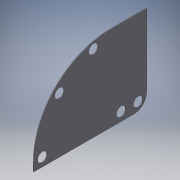
# Autodesk Inventor part: waterjet wall
Saved by Autodesk Inventor 2018 (Build 220112000, 112)
## iProperties
Created: 2020-01-24
Part Number: waterjet wall
Material: Generic
Document SubType Name: Modeling
Designer: s-2513225
Density: 1 g/cm^3
Appearance: Default
Author: s-2513225
Autodesk Inventor part; units mm, degrees
ref_plane "YZ Plane" through (0, 0, 0) normal (1, 0, 0) x (0, 1, 0)
ref_plane "XZ Plane" through (0, 0, 0) normal (0, 1, 0) x (-1, 0, 0)
ref_plane "XY Plane" through (0, 0, 0) normal (0, 0, 1) x (1, 0, 0)
sketch "Sketch1" plane through (0, 0, 0) normal (1, 0, 0) x (0, 1, 0)
  line L0 (-88.9, 0) -> (88.9, 0) construction
  line L1 (88.9, 0) -> (117.4115, 0) construction
  line L2 (165.1, -128.3993) -> (165.1, -77.5993)
  line L3 (-63.5, 151.0007) -> (-88.9, 151.0007)
  line L4 (-88.9, 151.0007) -> (-63.5, 151.0007) construction
  line L5 (-63.5, 151.0007) -> (-63.5, 125.6007) construction
  circle A0 centre (-63.5, 125.6007) radius 14.2875
  line L6 (-63.5, 125.6007) -> (-63.5, -26.7993) construction
  line L7 (-63.5, -26.7993) -> (139.7, -26.7993) construction
  circle A1 centre (139.7, -26.7993) radius 14.2875
  line L8 (-63.5, 125.6007) -> (76.2, 125.6007) construction
  line L9 (76.2, 125.6007) -> (76.2, 74.8007) construction
  circle A2 centre (76.2, 74.8007) radius 14.2875
  line L10 (-50.8, -185.5493) -> (165.1, -185.5493)
  line L11 (165.1, -185.5493) -> (165.1, -128.3993)
  arc A3 (165.1, -77.5993) -> (-63.5, 151.0007) centre (-63.5, -77.5993) ccw
  line L12 (-88.9, -147.4493) -> (-88.9, 151.0007)
  arc A4 (-88.9, -147.4493) -> (-50.8, -185.5493) centre (-50.8, -147.4493) ccw
  point P0 (0, 0)
  point P1 (165.1, 151.0007)
  point P2 (-88.9, -185.5493)
  dimension "d2" = 28.5115
  dimension "d5" = 279.4
  dimension "d8" = 25.4
  dimension "d9" = 25.4
  dimension "d10" = 28.575
  dimension "d11" = 152.4
  dimension "d12" = 203.2
  dimension "d13" = 28.575
  dimension "d14" = 139.7
  dimension "d15" = 50.8
  dimension "d16" = 28.575
  dimension "d22" = 254
  dimension "d34" = 228.6
  dimension "d35" = 38.1
  constraints: 26 end point, 5 centre point, 5 point on line, 4 perpendicular, 4 point on circle, 4 tangent, 3 coincident, 3 horizontal, 3 vertical, 1 parallel
  measures "d2" distance of L0.end L1.end
  measures "d5" distance of L2.start point (165.1, 151.001)
  measures "d8" distance of L3.end L4.end
  measures "d9" distance of L4.end L5.end
  measures "d10" diameter of A0
  measures "d11" distance of L6.start L6.end
  measures "d12" distance of L6.end L7.end
  measures "d13" diameter of A1
  measures "d14" distance of L6.start L8.end
  measures "d15" distance of L8.end L9.end
  measures "d16" diameter of A2
  measures "d22" distance of point (-88.9, -185.549) L10.end
  measures "d34" radius of A3
  measures "d35" radius of A4
extrude "Extrusion2" add sketch "Sketch1" along normal blind 1.778
sketch "Sketch2" plane through (1.778, 0, 0) normal (1, 0, 0) x (0, 0, -1)
  line L0 (185.5493, -50.8) -> (185.5493, 165.1) construction
  line L1 (160.1493, -88.9) -> (160.1493, -63.5) construction
  line L2 (160.1493, -63.5) -> (185.5493, -63.5) construction
  circle A0 centre (160.1493, -63.5) radius 14.2875
  line L3 (-151.0007, -88.9) -> (147.4493, -88.9) construction
  line L4 (160.1493, -88.9) -> (-151.0007, -88.9) construction
  line L5 (-151.0007, -88.9) -> (160.1493, -88.9) construction
  point P0 (0, 0)
  dimension "d24" = 25.4
  dimension "d25" = 28.575
  dimension "d36" = 311.15
  constraints: 8 end point, 1 centre point, 1 coincident, 1 collinear, 1 horizontal, 1 perpendicular
  measures "d24" distance of L1.start L1.end
  measures "d25" diameter of A0
  measures "d36" distance of L3.start L1.start
extrude "Extrusion3" cut sketch "Sketch2" against normal blind 1.778
sketch "Sketch3" plane through (0, 0, 0) normal (-1, 0, 0) x (0, 0, 1)
  line L0 (-185.5493, -88.9) -> (-134.7493, -88.9) construction
  line L1 (-134.7493, -88.9) -> (-109.3493, -88.9) construction
  line L2 (-109.3493, -88.9) -> (-109.3493, -63.5) construction
  circle A0 centre (-109.3493, -63.5) radius 14.2875
  point P0 (0, 0)
  dimension "d28" = 50.8
  dimension "d29" = 25.4
  dimension "d30" = 25.4
  dimension "d31" = 28.575
  constraints: 6 end point, 1 centre point, 1 coincident, 1 perpendicular
  measures "d28" distance of L0.start L0.end
  measures "d29" distance of L0.end L1.end
  measures "d30" distance of L1.end L2.end
  measures "d31" diameter of A0
extrude "Extrusion4" cut sketch "Sketch3" against normal blind 25.4
body "Solid2"
